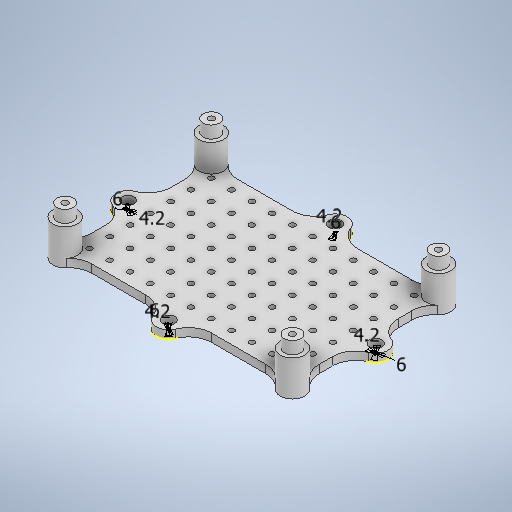
# Autodesk Inventor part: Bottom_Tip_Matrix
Saved by Autodesk Inventor 2025.1 (Build 291241000, 241)
## iProperties
Created: 2025-02-14
Part Number: Bottom_Tip_Matrix
Material: Generic
Document SubType Name: Modeling
Designer: m_kni
Density: 1 g/cm^3
Appearance: Default
Author: m_kni
Autodesk Inventor part; units mm, degrees
ref_plane "YZ Plane" through (0, 0, 0) normal (1, 0, 0) x (0, 1, 0)
ref_plane "XZ Plane" through (0, 0, 0) normal (0, 1, 0) x (-1, 0, 0)
ref_plane "XY Plane" through (0, 0, 0) normal (0, 0, 1) x (1, 0, 0)
sketch "Sketch1" plane through (0, 0, 0) normal (0, 1, 0) x (-1, 0, 0)
  line L0 (54.0633, -35.7627) -> (-55.9367, -35.7627)
  line L1 (-55.9367, -35.7627) -> (-55.9367, 36.2373)
  line L2 (-55.9367, 36.2373) -> (54.0633, 36.2373)
  line L3 (54.0633, -35.7627) -> (-55.9367, 36.2373) construction
  line L4 (-55.9367, -35.7627) -> (54.0633, 36.2373) construction
  circle A0 centre (-49.9367, 30.2373) radius 1.35
  circle A1 centre (-49.9367, 20.2373) radius 1.35
  circle A2 centre (-49.9367, 10.2373) radius 1.35
  circle A3 centre (-49.9367, 0.2373) radius 1.35
  circle A4 centre (-49.9367, -9.7627) radius 1.35
  circle A5 centre (-49.9367, -19.7627) radius 1.35
  circle A6 centre (-49.9367, -29.7627) radius 1.35
  circle A7 centre (-39.9367, 30.2373) radius 1.35
  circle A8 centre (-39.9367, 20.2373) radius 1.35
  circle A9 centre (-39.9367, 10.2373) radius 1.35
  circle A10 centre (-39.9367, 0.2373) radius 1.35
  circle A11 centre (-39.9367, -9.7627) radius 1.35
  circle A12 centre (-39.9367, -19.7627) radius 1.35
  circle A13 centre (-39.9367, -29.7627) radius 1.35
  circle A14 centre (-29.9367, 30.2373) radius 1.35
  circle A15 centre (-29.9367, 20.2373) radius 1.35
  circle A16 centre (-29.9367, 10.2373) radius 1.35
  circle A17 centre (-29.9367, 0.2373) radius 1.35
  circle A18 centre (-29.9367, -9.7627) radius 1.35
  circle A19 centre (-29.9367, -19.7627) radius 1.35
  circle A20 centre (-29.9367, -29.7627) radius 1.35
  circle A21 centre (-19.9367, 30.2373) radius 1.35
  circle A22 centre (-19.9367, 20.2373) radius 1.35
  circle A23 centre (-19.9367, 10.2373) radius 1.35
  circle A24 centre (-19.9367, 0.2373) radius 1.35
  circle A25 centre (-19.9367, -9.7627) radius 1.35
  circle A26 centre (-19.9367, -19.7627) radius 1.35
  circle A27 centre (-19.9367, -29.7627) radius 1.35
  circle A28 centre (-9.9367, 30.2373) radius 1.35
  circle A29 centre (-9.9367, 20.2373) radius 1.35
  circle A30 centre (-9.9367, 10.2373) radius 1.35
  circle A31 centre (-9.9367, 0.2373) radius 1.35
  circle A32 centre (-9.9367, -9.7627) radius 1.35
  circle A33 centre (-9.9367, -19.7627) radius 1.35
  circle A34 centre (-9.9367, -29.7627) radius 1.35
  circle A35 centre (0.0633, 30.2373) radius 1.35
  circle A36 centre (0.0633, 20.2373) radius 1.35
  circle A37 centre (0.0633, 10.2373) radius 1.35
  circle A38 centre (0.0633, 0.2373) radius 1.35
  circle A39 centre (0.0633, -9.7627) radius 1.35
  circle A40 centre (0.0633, -19.7627) radius 1.35
  circle A41 centre (0.0633, -29.7627) radius 1.35
  circle A42 centre (10.0633, 30.2373) radius 1.35
  circle A43 centre (10.0633, 20.2373) radius 1.35
  circle A44 centre (10.0633, 10.2373) radius 1.35
  circle A45 centre (10.0633, 0.2373) radius 1.35
  circle A46 centre (10.0633, -9.7627) radius 1.35
  circle A47 centre (10.0633, -19.7627) radius 1.35
  circle A48 centre (10.0633, -29.7627) radius 1.35
  circle A49 centre (20.0633, 30.2373) radius 1.35
  circle A50 centre (20.0633, 20.2373) radius 1.35
  circle A51 centre (20.0633, 10.2373) radius 1.35
  circle A52 centre (20.0633, 0.2373) radius 1.35
  circle A53 centre (20.0633, -9.7627) radius 1.35
  circle A54 centre (20.0633, -19.7627) radius 1.35
  circle A55 centre (20.0633, -29.7627) radius 1.35
  circle A56 centre (30.0633, 30.2373) radius 1.35
  circle A57 centre (30.0633, 20.2373) radius 1.35
  circle A58 centre (30.0633, 10.2373) radius 1.35
  circle A59 centre (30.0633, 0.2373) radius 1.35
  circle A60 centre (30.0633, -9.7627) radius 1.35
  circle A61 centre (30.0633, -19.7627) radius 1.35
  circle A62 centre (30.0633, -29.7627) radius 1.35
  circle A63 centre (40.0633, 30.2373) radius 1.35
  circle A64 centre (40.0633, 20.2373) radius 1.35
  circle A65 centre (40.0633, 10.2373) radius 1.35
  circle A66 centre (40.0633, 0.2373) radius 1.35
  circle A67 centre (40.0633, -9.7627) radius 1.35
  circle A68 centre (40.0633, -19.7627) radius 1.35
  circle A69 centre (40.0633, -29.7627) radius 1.35
  circle A70 centre (50.0633, 30.2373) radius 1.35
  circle A71 centre (50.0633, 20.2373) radius 1.35
  circle A72 centre (50.0633, 10.2373) radius 1.35
  circle A73 centre (50.0633, 0.2373) radius 1.35
  circle A74 centre (50.0633, -9.7627) radius 1.35
  circle A75 centre (50.0633, -19.7627) radius 1.35
  circle A76 centre (50.0633, -29.7627) radius 1.35
  line L5 (-55.9367, 36.2373) -> (56.0633, 36.2373)
  line L6 (56.0633, 36.2373) -> (56.0633, -35.7627)
  line L7 (56.0633, -35.7627) -> (-55.9367, -35.7627)
  line L8 (-55.9367, -35.7627) -> (-55.9367, 36.2373)
  circle A77 centre (-55.9367, 36.2373) radius 6
  circle A78 centre (-55.9367, -35.7627) radius 6
  circle A79 centre (56.0633, 36.2373) radius 6
  circle A80 centre (56.0633, -35.7627) radius 6
  point P0 (0, 0)
  point P1 (-0.9367, 0.2373)
  point P2 (56.0633, 30.2373)
  point P3 (-49.9367, -35.7627)
  point P4 (56.0633, -29.7627)
  point P5 (56.0633, 30.2373)
  point P6 (50.0633, 36.2373)
  point P7 (-49.9367, 36.2373)
  point P8 (-55.9367, 30.2373)
  point P9 (-55.9367, -29.7627)
  point P10 (-49.9367, -35.7627)
  point P11 (50.0633, -35.7627)
  dimension "d4" = 110
  dimension "d5" = 72
  dimension "d6" = 2.7
  dimension "d7" = 6
  dimension "d8" = 6
  dimension "d9" = 10
  dimension "d10" = 10
  dimension "d11" = 6
  dimension "d12" = 6
  dimension "d13" = 12
  dimension "d14" = 12
  dimension "d15" = 12
  dimension "d16" = 12
  constraints: 81 centre point, 18 end point, 5 coincident, 3 horizontal, 3 parallel, 2 midpoint, 2 perpendicular, 1 vertical, 152 other
  measures "d4" distance of L1.end L4.end
  measures "d5" distance of L1.start L1.end
  measures "d6" diameter of A0
  measures "d7" distance from line of A0.centre L2
  measures "d8" distance from line of A0.centre L1
  measures "d9" distance of A0.centre A1.centre
  measures "d10" distance of A0.centre A7.centre
  measures "d11" distance of point (56.063, 30.237) A70.centre
  measures "d12" distance of point (-49.937, -35.763) A6.centre
  measures "d13" diameter of A77
  measures "d14" diameter of A78
  measures "d15" diameter of A79
  measures "d16" diameter of A80
extrude "Extrusion1" add sketch "Sketch1" along normal blind 4
sketch "Sketch2" plane through (0, 4, 0) normal (0, 1, 0) x (1, 0, 0)
  arc A0 (49.9367, -36.2373) -> (55.9367, -30.2373) centre (55.9367, -36.2373) ccw projected
  arc A1 (-56.0633, -30.2373) -> (-50.0633, -36.2373) centre (-56.0633, -36.2373) ccw projected
  arc A2 (-50.0633, 35.7627) -> (-56.0633, 29.7627) centre (-56.0633, 35.7627) ccw projected
  arc A3 (55.9367, 29.7627) -> (49.9367, 35.7627) centre (55.9367, 35.7627) ccw projected
  circle A4 centre (-56.0633, -36.2373) radius 6
  circle A5 centre (-56.0633, 35.7627) radius 6
  circle A6 centre (55.9367, -36.2373) radius 6
  circle A7 centre (55.9367, 35.7627) radius 6
  point P0 (0, 0)
  point P1 (55.9367, 29.7627)
  point P2 (-56.0633, 29.7627)
  constraints: 4 coincident, 3 centre point, 3 concentric, 3 other
extrude "Extrusion2" add sketch "Sketch2" along normal blind 13.5
sketch "Sketch3" plane through (55.9367, 17.5, 36.2373) normal (0, 1, 0) x (1, 0, 0)
  circle A0 centre (0, 0) radius 4
  arc A1 (0, 66) -> (-6, 72) centre (0, 72) ccw projected
  circle A2 centre (0, 72) radius 4
  arc A3 (-112, 6) -> (-106, 0) centre (-112, 0) ccw projected
  circle A4 centre (-112, 0) radius 4
  circle A5 centre (-112, 72) radius 4
  point P0 (-55.9367, 36.2373)
  dimension "d21" = 8
  dimension "d22" = 8
  dimension "d23" = 8
  dimension "d24" = 8
  constraints: 4 centre point, 2 coincident
  measures "d21" diameter of A0
  measures "d22" diameter of A2
  measures "d23" diameter of A4
  measures "d24" diameter of A5
extrude "Extrusion3" add sketch "Sketch3" along normal blind 6
sketch "Sketch4" plane through (-56.0633, 23.5, 36.2373) normal (0, 1, 0) x (1, 0, 0)
  circle A0 centre (0, 0) radius 4 projected
  circle A1 centre (0, 72) radius 4 projected
  circle A2 centre (112, 0) radius 4 projected
  circle A3 centre (112, 72) radius 4 projected
  circle A4 centre (0, 0) radius 1.5
  circle A5 centre (112, 0) radius 1.5
  circle A6 centre (0, 72) radius 1.5
  circle A7 centre (112, 72) radius 1.5
  point P0 (56.0633, 36.2373)
  dimension "d27" = 3
  dimension "d28" = 3
  dimension "d29" = 3
  dimension "d30" = 3
  constraints: 4 centre point, 4 coincident
  measures "d27" diameter of A4
  measures "d28" diameter of A5
  measures "d29" diameter of A6
  measures "d30" diameter of A7
extrude "Extrusion4" cut sketch "Sketch4" against normal blind 8 contours A4 | A5 | A6 | A7
sketch "Sketch5" plane through (0, 4, 0) normal (0, 1, 0) x (1, 0, 0)
  line L0 (-50.0633, -36.2373) -> (49.9367, -36.2373) projected
  line L1 (-0.0633, -36.2373) -> (-0.0633, -41.2373)
  circle A0 centre (-0.0633, -41.2373) radius 6
  line L2 (49.9367, 35.7627) -> (-50.0633, 35.7627) projected
  line L3 (-56.0633, 29.7627) -> (-56.0633, -30.2373) projected
  line L4 (55.9367, -30.2373) -> (55.9367, 29.7627) projected
  circle A1 centre (60.9367, -0.2373) radius 6
  circle A2 centre (-0.0633, 40.7627) radius 6
  circle A3 centre (-61.0633, -0.2373) radius 6
  line L5 (60.9367, -6.2373) -> (55.9367, -6.2373)
  line L6 (60.9367, 5.7627) -> (55.9367, 5.7627)
  line L7 (-61.0633, 5.7627) -> (-56.0633, 5.7627)
  line L8 (-61.0633, -6.2373) -> (-56.0633, -6.2373)
  line L9 (-6.0633, -41.2373) -> (-6.0633, -36.2373)
  line L10 (5.9367, -41.2373) -> (5.9367, -36.2373)
  line L11 (-6.0633, 40.7627) -> (-6.0633, 35.7627)
  line L12 (5.9367, 40.7627) -> (5.9367, 35.7627)
  line L13 (-6.0633, -36.2373) -> (-5.0805, -36.2373)
  circle A4 centre (49.9367, -10.2373) radius 1.35 projected
  circle A5 centre (49.9367, -0.2373) radius 1.35 projected
  circle A6 centre (39.9367, -10.2373) radius 1.35 projected
  circle A7 centre (39.9367, -30.2373) radius 1.35 projected
  circle A8 centre (39.9367, -10.2373) radius 1.35 projected
  circle A9 centre (39.9367, 9.7627) radius 1.35 projected
  circle A10 centre (39.9367, 9.7627) radius 1.35 projected
  circle A11 centre (39.9367, 9.7627) radius 1.35 projected
  circle A12 centre (39.9367, 9.7627) radius 1.35 projected
  circle A13 centre (39.9367, 19.7627) radius 1.35 projected
  circle A14 centre (49.9367, 9.7627) radius 1.35 projected
  arc A15 (49.9367, -36.2373) -> (55.9367, -30.2373) centre (55.9367, -36.2373) ccw projected
  arc A16 (55.9367, -30.2373) -> (49.9367, -36.2373) centre (55.9367, -36.2373) ccw projected
  arc A17 (49.9367, 35.7627) -> (55.9367, 29.7627) centre (55.9367, 35.7627) ccw projected
  circle A18 centre (9.9367, 19.7627) radius 1.35 projected
  circle A19 centre (9.9367, 19.7627) radius 1.35 projected
  circle A20 centre (55.9367, 35.7627) radius 4 projected
  circle A21 centre (55.9367, 35.7627) radius 1.5 projected
  circle A22 centre (55.9367, 35.7627) radius 1.5 projected
  circle A23 centre (55.9367, 35.7627) radius 1.5 projected
  circle A24 centre (55.9367, 35.7627) radius 4 projected
  circle A25 centre (55.9367, 35.7627) radius 1.5 projected
  circle A26 centre (55.9367, 35.7627) radius 1.5 projected
  circle A27 centre (55.9367, 35.7627) radius 1.5 projected
  circle A28 centre (9.9367, 29.7627) radius 1.35 projected
  circle A29 centre (9.9367, 29.7627) radius 1.35 projected
  circle A30 centre (9.9367, 29.7627) radius 1.35 projected
  circle A31 centre (9.9367, 29.7627) radius 1.35 projected
  circle A32 centre (19.9367, 29.7627) radius 1.35 projected
  circle A33 centre (19.9367, 29.7627) radius 1.35 projected
  circle A34 centre (19.9367, 9.7627) radius 1.35 projected
  circle A35 centre (19.9367, 9.7627) radius 1.35 projected
  circle A36 centre (19.9367, 9.7627) radius 1.35 projected
  circle A37 centre (19.9367, 9.7627) radius 1.35 projected
  circle A38 centre (19.9367, 19.7627) radius 1.35 projected
  circle A39 centre (19.9367, 19.7627) radius 1.35 projected
  circle A40 centre (19.9367, 19.7627) radius 1.35 projected
  circle A41 centre (19.9367, 29.7627) radius 1.35 projected
  circle A42 centre (19.9367, 29.7627) radius 1.35 projected
  circle A43 centre (9.9367, 9.7627) radius 1.35 projected
  circle A44 centre (9.9367, 9.7627) radius 1.35 projected
  circle A45 centre (9.9367, 19.7627) radius 1.35 projected
  circle A46 centre (9.9367, 19.7627) radius 1.35 projected
  circle A47 centre (9.9367, 9.7627) radius 1.35 projected
  circle A48 centre (19.9367, 19.7627) radius 1.35 projected
  circle A49 centre (29.9367, 29.7627) radius 1.35 projected
  arc A50 (55.9367, 29.7627) -> (49.9367, 35.7627) centre (55.9367, 35.7627) ccw projected
  circle A51 centre (29.9367, 9.7627) radius 1.35 projected
  circle A52 centre (-0.0633, -0.2373) radius 1.35 projected
  circle A53 centre (-0.0633, -0.2373) radius 1.35 projected
  circle A54 centre (-0.0633, -10.2373) radius 1.35 projected
  circle A55 centre (-10.0633, -10.2373) radius 1.35 projected
  circle A56 centre (-10.0633, -10.2373) radius 1.35 projected
  circle A57 centre (55.9367, -36.2373) radius 1.5 projected
  circle A58 centre (49.9367, 9.7627) radius 1.35 projected
  circle A59 centre (49.9367, 9.7627) radius 1.35 projected
  circle A60 centre (55.9367, -36.2373) radius 4 projected
  circle A61 centre (49.9367, 19.7627) radius 1.35 projected
  circle A62 centre (49.9367, 19.7627) radius 1.35 projected
  circle A63 centre (-0.0633, 9.7627) radius 1.35 projected
  circle A64 centre (-10.0633, 9.7627) radius 1.35 projected
  circle A65 centre (-10.0633, 9.7627) radius 1.35 projected
  circle A66 centre (-0.0633, 9.7627) radius 1.35 projected
  circle A67 centre (-0.0633, -20.2373) radius 1.35 projected
  circle A68 centre (-0.0633, -20.2373) radius 1.35 projected
  circle A69 centre (19.9367, -20.2373) radius 1.35 projected
  circle A70 centre (9.9367, -30.2373) radius 1.35 projected
  circle A71 centre (-0.0633, -30.2373) radius 1.35 projected
  circle A72 centre (-0.0633, -30.2373) radius 1.35 projected
  circle A73 centre (-10.0633, -20.2373) radius 1.35 projected
  circle A74 centre (-10.0633, -20.2373) radius 1.35 projected
  circle A75 centre (19.9367, -20.2373) radius 1.35 projected
  circle A76 centre (9.9367, -0.2373) radius 1.35 projected
  circle A77 centre (-10.0633, -30.2373) radius 1.35 projected
  circle A78 centre (-10.0633, -30.2373) radius 1.35 projected
  circle A79 centre (9.9367, -0.2373) radius 1.35 projected
  circle A80 centre (-0.0633, 19.7627) radius 1.35 projected
  circle A81 centre (-0.0633, 19.7627) radius 1.35 projected
  circle A82 centre (-0.0633, 29.7627) radius 1.35 projected
  circle A83 centre (-0.0633, 29.7627) radius 1.35 projected
  circle A84 centre (-10.0633, 19.7627) radius 1.35 projected
  circle A85 centre (-10.0633, 19.7627) radius 1.35 projected
  circle A86 centre (-0.0633, 19.7627) radius 1.35 projected
  circle A87 centre (-0.0633, 19.7627) radius 1.35 projected
  circle A88 centre (-0.0633, 29.7627) radius 1.35 projected
  circle A89 centre (-0.0633, 29.7627) radius 1.35 projected
  circle A90 centre (-10.0633, -0.2373) radius 1.35 projected
  circle A91 centre (-10.0633, -0.2373) radius 1.35 projected
  circle A92 centre (55.9367, -36.2373) radius 4 projected
  circle A93 centre (55.9367, -36.2373) radius 1.5 projected
  circle A94 centre (55.9367, -36.2373) radius 1.5 projected
  circle A95 centre (55.9367, -36.2373) radius 4 projected
  circle A96 centre (55.9367, -36.2373) radius 1.5 projected
  circle A97 centre (55.9367, -36.2373) radius 1.5 projected
  circle A98 centre (39.9367, -30.2373) radius 1.35 projected
  circle A99 centre (39.9367, -30.2373) radius 1.35 projected
  circle A100 centre (39.9367, -0.2373) radius 1.35 projected
  circle A101 centre (39.9367, -0.2373) radius 1.35 projected
  circle A102 centre (39.9367, -10.2373) radius 1.35 projected
  circle A103 centre (39.9367, -10.2373) radius 1.35 projected
  circle A104 centre (39.9367, -20.2373) radius 1.35 projected
  circle A105 centre (39.9367, -20.2373) radius 1.35 projected
  circle A106 centre (49.9367, -20.2373) radius 1.35 projected
  circle A107 centre (49.9367, -20.2373) radius 1.35 projected
  circle A108 centre (49.9367, -10.2373) radius 1.35 projected
  circle A109 centre (49.9367, -10.2373) radius 1.35 projected
  circle A110 centre (49.9367, -30.2373) radius 1.35 projected
  circle A111 centre (49.9367, -30.2373) radius 1.35 projected
  circle A112 centre (55.9367, -36.2373) radius 4 projected
  circle A113 centre (55.9367, -36.2373) radius 4 projected
  circle A114 centre (55.9367, -36.2373) radius 6 projected
  circle A115 centre (55.9367, -36.2373) radius 6 projected
  arc A116 (49.9367, -36.2373) -> (55.9367, -30.2373) centre (55.9367, -36.2373) ccw projected
  arc A117 (55.9367, -30.2373) -> (49.9367, -36.2373) centre (55.9367, -36.2373) ccw projected
  circle A118 centre (55.9367, -36.2373) radius 4 projected
  circle A119 centre (55.9367, -36.2373) radius 6 projected
  line L14 (55.9367, -30.2373) -> (55.9367, 29.7627) projected
  line L15 (55.9367, -30.2373) -> (55.9367, 29.7627) projected
  circle A120 centre (49.9367, -0.2373) radius 1.35 projected
  circle A121 centre (49.9367, -0.2373) radius 1.35 projected
  circle A122 centre (-20.0633, 19.7627) radius 1.35 projected
  circle A123 centre (-20.0633, 29.7627) radius 1.35 projected
  circle A124 centre (-20.0633, 29.7627) radius 1.35 projected
  circle A125 centre (-20.0633, 19.7627) radius 1.35 projected
  circle A126 centre (-40.0633, -20.2373) radius 1.35 projected
  circle A127 centre (-40.0633, -20.2373) radius 1.35 projected
  circle A128 centre (-40.0633, -30.2373) radius 1.35 projected
  circle A129 centre (-40.0633, -30.2373) radius 1.35 projected
  circle A130 centre (-30.0633, -20.2373) radius 1.35 projected
  circle A131 centre (-30.0633, -20.2373) radius 1.35 projected
  circle A132 centre (-20.0633, 9.7627) radius 1.35 projected
  circle A133 centre (-20.0633, 9.7627) radius 1.35 projected
  circle A134 centre (-30.0633, -0.2373) radius 1.35 projected
  circle A135 centre (-30.0633, -0.2373) radius 1.35 projected
  circle A136 centre (-20.0633, -30.2373) radius 1.35 projected
  circle A137 centre (-20.0633, -30.2373) radius 1.35 projected
  circle A138 centre (-20.0633, -10.2373) radius 1.35 projected
  circle A139 centre (-20.0633, -10.2373) radius 1.35 projected
  circle A140 centre (-20.0633, -0.2373) radius 1.35 projected
  circle A141 centre (-20.0633, -0.2373) radius 1.35 projected
  circle A142 centre (-30.0633, 9.7627) radius 1.35 projected
  circle A143 centre (-20.0633, -20.2373) radius 1.35 projected
  circle A144 centre (-20.0633, -20.2373) radius 1.35 projected
  circle A145 centre (-30.0633, -10.2373) radius 1.35 projected
  circle A146 centre (-30.0633, -10.2373) radius 1.35 projected
  circle A147 centre (-40.0633, -10.2373) radius 1.35 projected
  circle A148 centre (-30.0633, -30.2373) radius 1.35 projected
  circle A149 centre (-30.0633, -30.2373) radius 1.35 projected
  circle A150 centre (-30.0633, 9.7627) radius 1.35 projected
  circle A151 centre (-40.0633, -0.2373) radius 1.35 projected
  circle A152 centre (-40.0633, -0.2373) radius 1.35 projected
  circle A153 centre (-50.0633, 19.7627) radius 1.35 projected
  circle A154 centre (-50.0633, 19.7627) radius 1.35 projected
  circle A155 centre (-50.0633, 9.7627) radius 1.35 projected
  circle A156 centre (-50.0633, 9.7627) radius 1.35 projected
  circle A157 centre (-40.0633, 19.7627) radius 1.35 projected
  circle A158 centre (-40.0633, 19.7627) radius 1.35 projected
  circle A159 centre (-50.0633, -10.2373) radius 1.35 projected
  circle A160 centre (-30.0633, 19.7627) radius 1.35 projected
  circle A161 centre (-30.0633, 29.7627) radius 1.35 projected
  circle A162 centre (-30.0633, 29.7627) radius 1.35 projected
  circle A163 centre (-50.0633, -10.2373) radius 1.35 projected
  circle A164 centre (-30.0633, 19.7627) radius 1.35 projected
  circle A165 centre (-56.0633, -36.2373) radius 1.5 projected
  circle A166 centre (-56.0633, -36.2373) radius 1.5 projected
  circle A167 centre (-56.0633, -36.2373) radius 1.5 projected
  circle A168 centre (-56.0633, -36.2373) radius 1.5 projected
  circle A169 centre (-56.0633, -36.2373) radius 1.5 projected
  arc A170 (-50.0633, -36.2373) -> (-56.0633, -30.2373) centre (-56.0633, -36.2373) ccw projected
  arc A171 (-56.0633, -30.2373) -> (-50.0633, -36.2373) centre (-56.0633, -36.2373) ccw projected
  line L16 (-56.0633, 29.7627) -> (-56.0633, -30.2373) projected
  arc A172 (-56.0633, 29.7627) -> (-50.0633, 35.7627) centre (-56.0633, 35.7627) ccw projected
  arc A173 (-50.0633, 35.7627) -> (-56.0633, 29.7627) centre (-56.0633, 35.7627) ccw projected
  circle A174 centre (-56.0633, 35.7627) radius 4 projected
  circle A175 centre (-56.0633, 35.7627) radius 1.5 projected
  circle A176 centre (-56.0633, 35.7627) radius 1.5 projected
  circle A177 centre (-56.0633, 35.7627) radius 1.5 projected
  circle A178 centre (-56.0633, 35.7627) radius 4 projected
  circle A179 centre (-56.0633, 35.7627) radius 1.5 projected
  circle A180 centre (-56.0633, 35.7627) radius 1.5 projected
  circle A181 centre (-56.0633, 35.7627) radius 6 projected
  arc A182 (-50.0633, 35.7627) -> (-56.0633, 29.7627) centre (-56.0633, 35.7627) ccw projected
  arc A183 (-56.0633, 29.7627) -> (-50.0633, 35.7627) centre (-56.0633, 35.7627) ccw projected
  circle A184 centre (-50.0633, 19.7627) radius 1.35 projected
  circle A185 centre (-50.0633, 19.7627) radius 1.35 projected
  circle A186 centre (-50.0633, 9.7627) radius 1.35 projected
  circle A187 centre (-50.0633, 9.7627) radius 1.35 projected
  circle A188 centre (-40.0633, 19.7627) radius 1.35 projected
  circle A189 centre (-40.0633, 19.7627) radius 1.35 projected
  circle A190 centre (-10.0633, 9.7627) radius 1.35 projected
  circle A191 centre (-10.0633, 9.7627) radius 1.35 projected
  circle A192 centre (-30.0633, 9.7627) radius 1.35 projected
  circle A193 centre (-30.0633, 9.7627) radius 1.35 projected
  circle A194 centre (-40.0633, 9.7627) radius 1.35 projected
  circle A195 centre (-40.0633, 9.7627) radius 1.35 projected
  circle A196 centre (-30.0633, 19.7627) radius 1.35 projected
  circle A197 centre (-30.0633, 19.7627) radius 1.35 projected
  circle A198 centre (-56.0633, 35.7627) radius 4 projected
  circle A199 centre (-56.0633, 35.7627) radius 4 projected
  circle A200 centre (-56.0633, 35.7627) radius 4 projected
  circle A201 centre (-56.0633, 35.7627) radius 6 projected
  circle A202 centre (-50.0633, 29.7627) radius 1.35 projected
  circle A203 centre (-50.0633, 29.7627) radius 1.35 projected
  circle A204 centre (-20.0633, 19.7627) radius 1.35 projected
  circle A205 centre (-20.0633, 19.7627) radius 1.35 projected
  circle A206 centre (-40.0633, 29.7627) radius 1.35 projected
  circle A207 centre (-40.0633, 29.7627) radius 1.35 projected
  circle A208 centre (-30.0633, 29.7627) radius 1.35 projected
  circle A209 centre (-30.0633, 29.7627) radius 1.35 projected
  circle A210 centre (-10.0633, 19.7627) radius 1.35 projected
  circle A211 centre (-10.0633, 19.7627) radius 1.35 projected
  circle A212 centre (-20.0633, 29.7627) radius 1.35 projected
  circle A213 centre (-20.0633, 29.7627) radius 1.35 projected
  circle A214 centre (-10.0633, 29.7627) radius 1.35 projected
  circle A215 centre (-10.0633, 29.7627) radius 1.35 projected
  circle A216 centre (-20.0633, 9.7627) radius 1.35 projected
  circle A217 centre (-20.0633, 9.7627) radius 1.35 projected
  circle A218 centre (-56.0633, -36.2373) radius 4 projected
  circle A219 centre (-56.0633, -36.2373) radius 1.5 projected
  circle A220 centre (-56.0633, -36.2373) radius 4 projected
  circle A221 centre (-56.0633, -36.2373) radius 4 projected
  circle A222 centre (-56.0633, -36.2373) radius 6 projected
  arc A223 (-56.0633, -30.2373) -> (-50.0633, -36.2373) centre (-56.0633, -36.2373) ccw projected
  arc A224 (-50.0633, -36.2373) -> (-56.0633, -30.2373) centre (-56.0633, -36.2373) ccw projected
  line L17 (-56.0633, 29.7627) -> (-56.0633, -30.2373) projected
  line L18 (-56.0633, 29.7627) -> (-56.0633, -30.2373) projected
  circle A225 centre (-40.0633, -0.2373) radius 1.35 projected
  circle A226 centre (-40.0633, -0.2373) radius 1.35 projected
  circle A227 centre (-50.0633, -10.2373) radius 1.35 projected
  circle A228 centre (-50.0633, -10.2373) radius 1.35 projected
  circle A229 centre (-40.0633, -20.2373) radius 1.35 projected
  circle A230 centre (-40.0633, -20.2373) radius 1.35 projected
  circle A231 centre (-40.0633, -30.2373) radius 1.35 projected
  circle A232 centre (-40.0633, -30.2373) radius 1.35 projected
  circle A233 centre (-30.0633, -20.2373) radius 1.35 projected
  circle A234 centre (-30.0633, -20.2373) radius 1.35 projected
  circle A235 centre (-30.0633, -0.2373) radius 1.35 projected
  circle A236 centre (-30.0633, -0.2373) radius 1.35 projected
  circle A237 centre (-10.0633, -0.2373) radius 1.35 projected
  circle A238 centre (-10.0633, -0.2373) radius 1.35 projected
  circle A239 centre (-20.0633, -0.2373) radius 1.35 projected
  circle A240 centre (-20.0633, -0.2373) radius 1.35 projected
  circle A241 centre (-50.0633, -0.2373) radius 1.35 projected
  circle A242 centre (-50.0633, -0.2373) radius 1.35 projected
  circle A243 centre (-20.0633, -10.2373) radius 1.35 projected
  circle A244 centre (-20.0633, -10.2373) radius 1.35 projected
  circle A245 centre (-10.0633, -10.2373) radius 1.35 projected
  circle A246 centre (-10.0633, -10.2373) radius 1.35 projected
  circle A247 centre (-40.0633, -10.2373) radius 1.35 projected
  circle A248 centre (-40.0633, -10.2373) radius 1.35 projected
  circle A249 centre (-10.0633, -20.2373) radius 1.35 projected
  circle A250 centre (-10.0633, -20.2373) radius 1.35 projected
  circle A251 centre (-20.0633, -20.2373) radius 1.35 projected
  circle A252 centre (-20.0633, -20.2373) radius 1.35 projected
  circle A253 centre (-10.0633, -30.2373) radius 1.35 projected
  circle A254 centre (-10.0633, -30.2373) radius 1.35 projected
  circle A255 centre (-20.0633, -30.2373) radius 1.35 projected
  circle A256 centre (-20.0633, -30.2373) radius 1.35 projected
  circle A257 centre (-30.0633, -30.2373) radius 1.35 projected
  circle A258 centre (-30.0633, -30.2373) radius 1.35 projected
  circle A259 centre (-50.0633, -20.2373) radius 1.35 projected
  circle A260 centre (-50.0633, -20.2373) radius 1.35 projected
  circle A261 centre (-50.0633, -30.2373) radius 1.35 projected
  circle A262 centre (-50.0633, -30.2373) radius 1.35 projected
  circle A263 centre (-56.0633, -36.2373) radius 4 projected
  circle A264 centre (-56.0633, -36.2373) radius 4 projected
  circle A265 centre (-56.0633, -36.2373) radius 4 projected
  circle A266 centre (-56.0633, -36.2373) radius 6 projected
  circle A267 centre (-30.0633, -10.2373) radius 1.35 projected
  circle A268 centre (-30.0633, -10.2373) radius 1.35 projected
  circle A269 centre (-40.0633, -10.2373) radius 1.35 projected
  circle A270 centre (-40.0633, 29.7627) radius 1.35 projected
  circle A271 centre (-40.0633, 29.7627) radius 1.35 projected
  circle A272 centre (-40.0633, 9.7627) radius 1.35 projected
  circle A273 centre (-50.0633, 29.7627) radius 1.35 projected
  circle A274 centre (-50.0633, 29.7627) radius 1.35 projected
  circle A275 centre (-56.0633, 35.7627) radius 4 projected
  circle A276 centre (-56.0633, 35.7627) radius 6 projected
  circle A277 centre (-50.0633, -0.2373) radius 1.35 projected
  circle A278 centre (-50.0633, -0.2373) radius 1.35 projected
  circle A279 centre (-50.0633, -20.2373) radius 1.35 projected
  circle A280 centre (-50.0633, -20.2373) radius 1.35 projected
  circle A281 centre (-50.0633, -30.2373) radius 1.35 projected
  circle A282 centre (-50.0633, -30.2373) radius 1.35 projected
  circle A283 centre (-56.0633, -36.2373) radius 6 projected
  circle A284 centre (-40.0633, 9.7627) radius 1.35 projected
  circle A285 centre (29.9367, 29.7627) radius 1.35 projected
  circle A286 centre (49.9367, -0.2373) radius 1.35 projected
  circle A287 centre (29.9367, 9.7627) radius 1.35 projected
  circle A288 centre (29.9367, 9.7627) radius 1.35 projected
  circle A289 centre (29.9367, 9.7627) radius 1.35 projected
  circle A290 centre (39.9367, -0.2373) radius 1.35 projected
  circle A291 centre (39.9367, -0.2373) radius 1.35 projected
  circle A292 centre (29.9367, -0.2373) radius 1.35 projected
  circle A293 centre (49.9367, -10.2373) radius 1.35 projected
  circle A294 centre (29.9367, -0.2373) radius 1.35 projected
  circle A295 centre (19.9367, -0.2373) radius 1.35 projected
  circle A296 centre (19.9367, -0.2373) radius 1.35 projected
  circle A297 centre (19.9367, -10.2373) radius 1.35 projected
  circle A298 centre (19.9367, -10.2373) radius 1.35 projected
  line L19 (55.9367, -30.2373) -> (55.9367, 29.7627) projected
  circle A299 centre (-10.0633, 29.7627) radius 1.35 projected
  circle A300 centre (-10.0633, 29.7627) radius 1.35 projected
  circle A301 centre (55.9367, -36.2373) radius 1.5 projected
  circle A302 centre (29.9367, -30.2373) radius 1.35 projected
  circle A303 centre (29.9367, -30.2373) radius 1.35 projected
  circle A304 centre (19.9367, -30.2373) radius 1.35 projected
  line L20 (49.9367, 35.7627) -> (-50.0633, 35.7627) projected
  line L21 (49.9367, 35.7627) -> (-50.0633, 35.7627) projected
  line L22 (49.9367, 35.7627) -> (-50.0633, 35.7627) projected
  circle A305 centre (-56.0633, 35.7627) radius 1.5 projected
  line L23 (-50.0633, -36.2373) -> (49.9367, -36.2373) projected
  line L24 (-50.0633, -36.2373) -> (49.9367, -36.2373) projected
  line L25 (-50.0633, -36.2373) -> (49.9367, -36.2373) projected
  arc A306 (55.9367, -30.2373) -> (49.9367, -36.2373) centre (55.9367, -36.2373) ccw projected
  line L26 (55.9367, -30.2373) -> (55.9367, 29.7627) projected
  arc A307 (49.9367, 35.7627) -> (55.9367, 29.7627) centre (55.9367, 35.7627) ccw projected
  line L27 (49.9367, 35.7627) -> (-50.0633, 35.7627) projected
  arc A308 (-56.0633, 29.7627) -> (-50.0633, 35.7627) centre (-56.0633, 35.7627) ccw projected
  line L28 (-56.0633, 29.7627) -> (-56.0633, -30.2373) projected
  arc A309 (-50.0633, -36.2373) -> (-56.0633, -30.2373) centre (-56.0633, -36.2373) ccw projected
  line L29 (-50.0633, -36.2373) -> (49.9367, -36.2373) projected
  circle A310 centre (-40.0633, -0.2373) radius 1.35 projected
  circle A311 centre (-50.0633, 19.7627) radius 1.35 projected
  circle A312 centre (-50.0633, 9.7627) radius 1.35 projected
  circle A313 centre (-40.0633, 19.7627) radius 1.35 projected
  circle A314 centre (-50.0633, -10.2373) radius 1.35 projected
  circle A315 centre (-40.0633, -20.2373) radius 1.35 projected
  circle A316 centre (-40.0633, -30.2373) radius 1.35 projected
  circle A317 centre (-30.0633, -20.2373) radius 1.35 projected
  circle A318 centre (-30.0633, 19.7627) radius 1.35 projected
  circle A319 centre (-30.0633, 29.7627) radius 1.35 projected
  circle A320 centre (-20.0633, 9.7627) radius 1.35 projected
  circle A321 centre (-30.0633, -0.2373) radius 1.35 projected
  circle A322 centre (-20.0633, -30.2373) radius 1.35 projected
  circle A323 centre (-20.0633, -10.2373) radius 1.35 projected
  circle A324 centre (9.9367, 29.7627) radius 1.35 projected
  circle A325 centre (29.9367, -10.2373) radius 1.35 projected
  circle A326 centre (29.9367, -30.2373) radius 1.35 projected
  circle A327 centre (19.9367, -0.2373) radius 1.35 projected
  circle A328 centre (19.9367, -10.2373) radius 1.35 projected
  circle A329 centre (29.9367, 29.7627) radius 1.35 projected
  circle A330 centre (19.9367, 29.7627) radius 1.35 projected
  circle A331 centre (19.9367, 9.7627) radius 1.35 projected
  circle A332 centre (9.9367, -20.2373) radius 1.35 projected
  circle A333 centre (9.9367, -10.2373) radius 1.35 projected
  circle A334 centre (-0.0633, 19.7627) radius 1.35 projected
  circle A335 centre (-0.0633, 29.7627) radius 1.35 projected
  circle A336 centre (-10.0633, 29.7627) radius 1.35 projected
  circle A337 centre (-10.0633, -30.2373) radius 1.35 projected
  circle A338 centre (39.9367, -30.2373) radius 1.35 projected
  circle A339 centre (49.9367, -20.2373) radius 1.35 projected
  circle A340 centre (9.9367, -0.2373) radius 1.35 projected
  circle A341 centre (-10.0633, 9.7627) radius 1.35 projected
  circle A342 centre (-0.0633, 9.7627) radius 1.35 projected
  circle A343 centre (19.9367, -30.2373) radius 1.35 projected
  circle A344 centre (49.9367, -10.2373) radius 1.35 projected
  circle A345 centre (29.9367, -0.2373) radius 1.35 projected
  circle A346 centre (49.9367, -0.2373) radius 1.35 projected
  circle A347 centre (39.9367, -0.2373) radius 1.35 projected
  circle A348 centre (49.9367, 9.7627) radius 1.35 projected
  circle A349 centre (39.9367, 9.7627) radius 1.35 projected
  circle A350 centre (49.9367, 19.7627) radius 1.35 projected
  circle A351 centre (39.9367, 29.7627) radius 1.35 projected
  circle A352 centre (-0.0633, -0.2373) radius 1.35 projected
  circle A353 centre (-10.0633, -10.2373) radius 1.35 projected
  circle A354 centre (39.9367, 19.7627) radius 1.35 projected
  circle A355 centre (39.9367, -20.2373) radius 1.35 projected
  circle A356 centre (-10.0633, -20.2373) radius 1.35 projected
  circle A357 centre (-10.0633, 19.7627) radius 1.35 projected
  circle A358 centre (-10.0633, -0.2373) radius 1.35 projected
  circle A359 centre (-0.0633, -20.2373) radius 1.35 projected
  circle A360 centre (-0.0633, -30.2373) radius 1.35 projected
  circle A361 centre (-0.0633, -10.2373) radius 1.35 projected
  circle A362 centre (29.9367, 9.7627) radius 1.35 projected
  circle A363 centre (19.9367, 19.7627) radius 1.35 projected
  circle A364 centre (29.9367, 19.7627) radius 1.35 projected
  circle A365 centre (9.9367, -30.2373) radius 1.35 projected
  circle A366 centre (19.9367, -20.2373) radius 1.35 projected
  circle A367 centre (29.9367, -20.2373) radius 1.35 projected
  circle A368 centre (39.9367, -10.2373) radius 1.35 projected
  circle A369 centre (9.9367, 19.7627) radius 1.35 projected
  circle A370 centre (9.9367, 9.7627) radius 1.35 projected
  circle A371 centre (-20.0633, -20.2373) radius 1.35 projected
  circle A372 centre (-20.0633, -0.2373) radius 1.35 projected
  circle A373 centre (-30.0633, 9.7627) radius 1.35 projected
  circle A374 centre (-20.0633, 19.7627) radius 1.35 projected
  circle A375 centre (-20.0633, 29.7627) radius 1.35 projected
  circle A376 centre (-30.0633, -10.2373) radius 1.35 projected
  circle A377 centre (-30.0633, -30.2373) radius 1.35 projected
  circle A378 centre (-40.0633, -10.2373) radius 1.35 projected
  circle A379 centre (-50.0633, -20.2373) radius 1.35 projected
  circle A380 centre (-40.0633, 29.7627) radius 1.35 projected
  circle A381 centre (-40.0633, 9.7627) radius 1.35 projected
  circle A382 centre (-50.0633, -0.2373) radius 1.35 projected
  circle A383 centre (-50.0633, 29.7627) radius 1.35 projected
  circle A384 centre (-50.0633, -30.2373) radius 1.35 projected
  circle A385 centre (49.9367, -30.2373) radius 1.35 projected
  circle A386 centre (49.9367, 29.7627) radius 1.35 projected
  arc A387 (-56.0633, -30.2373) -> (-50.0633, -36.2373) centre (-56.0633, -36.2373) ccw projected
  line L30 (-56.0633, 29.7627) -> (-56.0633, -30.2373) projected
  arc A388 (-50.0633, 35.7627) -> (-56.0633, 29.7627) centre (-56.0633, 35.7627) ccw projected
  line L31 (49.9367, 35.7627) -> (-50.0633, 35.7627) projected
  arc A389 (55.9367, 29.7627) -> (49.9367, 35.7627) centre (55.9367, 35.7627) ccw projected
  line L32 (55.9367, -30.2373) -> (55.9367, 29.7627) projected
  arc A390 (49.9367, -36.2373) -> (55.9367, -30.2373) centre (55.9367, -36.2373) ccw projected
  line L33 (-50.0633, -36.2373) -> (49.9367, -36.2373) projected
  circle A391 centre (-40.0633, -0.2373) radius 1.35 projected
  circle A392 centre (-50.0633, 19.7627) radius 1.35 projected
  circle A393 centre (-50.0633, 9.7627) radius 1.35 projected
  circle A394 centre (-40.0633, 19.7627) radius 1.35 projected
  circle A395 centre (-50.0633, -10.2373) radius 1.35 projected
  circle A396 centre (-40.0633, -20.2373) radius 1.35 projected
  circle A397 centre (-40.0633, -30.2373) radius 1.35 projected
  circle A398 centre (-30.0633, -20.2373) radius 1.35 projected
  circle A399 centre (-30.0633, 19.7627) radius 1.35 projected
  circle A400 centre (-30.0633, 29.7627) radius 1.35 projected
  circle A401 centre (-20.0633, 9.7627) radius 1.35 projected
  circle A402 centre (-30.0633, -0.2373) radius 1.35 projected
  circle A403 centre (-20.0633, -30.2373) radius 1.35 projected
  circle A404 centre (-20.0633, -10.2373) radius 1.35 projected
  circle A405 centre (9.9367, 29.7627) radius 1.35 projected
  circle A406 centre (29.9367, -10.2373) radius 1.35 projected
  circle A407 centre (29.9367, -30.2373) radius 1.35 projected
  circle A408 centre (19.9367, -0.2373) radius 1.35 projected
  circle A409 centre (19.9367, -10.2373) radius 1.35 projected
  circle A410 centre (29.9367, 29.7627) radius 1.35 projected
  circle A411 centre (19.9367, 29.7627) radius 1.35 projected
  circle A412 centre (19.9367, 9.7627) radius 1.35 projected
  circle A413 centre (9.9367, -20.2373) radius 1.35 projected
  circle A414 centre (9.9367, -10.2373) radius 1.35 projected
  circle A415 centre (-0.0633, 19.7627) radius 1.35 projected
  circle A416 centre (-0.0633, 29.7627) radius 1.35 projected
  circle A417 centre (-10.0633, 29.7627) radius 1.35 projected
  circle A418 centre (-10.0633, -30.2373) radius 1.35 projected
  circle A419 centre (39.9367, -30.2373) radius 1.35 projected
  circle A420 centre (49.9367, -20.2373) radius 1.35 projected
  circle A421 centre (9.9367, -0.2373) radius 1.35 projected
  circle A422 centre (-10.0633, 9.7627) radius 1.35 projected
  circle A423 centre (-0.0633, 9.7627) radius 1.35 projected
  circle A424 centre (19.9367, -30.2373) radius 1.35 projected
  circle A425 centre (49.9367, -10.2373) radius 1.35 projected
  circle A426 centre (29.9367, -0.2373) radius 1.35 projected
  circle A427 centre (49.9367, -0.2373) radius 1.35 projected
  circle A428 centre (39.9367, -0.2373) radius 1.35 projected
  circle A429 centre (49.9367, 9.7627) radius 1.35 projected
  circle A430 centre (39.9367, 9.7627) radius 1.35 projected
  circle A431 centre (49.9367, 19.7627) radius 1.35 projected
  circle A432 centre (39.9367, 29.7627) radius 1.35 projected
  circle A433 centre (-0.0633, -0.2373) radius 1.35 projected
  circle A434 centre (-10.0633, -10.2373) radius 1.35 projected
  circle A435 centre (39.9367, 19.7627) radius 1.35 projected
  circle A436 centre (39.9367, -20.2373) radius 1.35 projected
  circle A437 centre (-10.0633, -20.2373) radius 1.35 projected
  circle A438 centre (-10.0633, 19.7627) radius 1.35 projected
  circle A439 centre (-10.0633, -0.2373) radius 1.35 projected
  circle A440 centre (-0.0633, -20.2373) radius 1.35 projected
  circle A441 centre (-0.0633, -30.2373) radius 1.35 projected
  circle A442 centre (-0.0633, -10.2373) radius 1.35 projected
  circle A443 centre (29.9367, 9.7627) radius 1.35 projected
  circle A444 centre (19.9367, 19.7627) radius 1.35 projected
  circle A445 centre (29.9367, 19.7627) radius 1.35 projected
  circle A446 centre (9.9367, -30.2373) radius 1.35 projected
  circle A447 centre (19.9367, -20.2373) radius 1.35 projected
  circle A448 centre (29.9367, -20.2373) radius 1.35 projected
  circle A449 centre (39.9367, -10.2373) radius 1.35 projected
  circle A450 centre (9.9367, 19.7627) radius 1.35 projected
  circle A451 centre (9.9367, 9.7627) radius 1.35 projected
  circle A452 centre (-20.0633, -20.2373) radius 1.35 projected
  circle A453 centre (-20.0633, -0.2373) radius 1.35 projected
  circle A454 centre (-30.0633, 9.7627) radius 1.35 projected
  circle A455 centre (-20.0633, 19.7627) radius 1.35 projected
  circle A456 centre (-20.0633, 29.7627) radius 1.35 projected
  circle A457 centre (-30.0633, -10.2373) radius 1.35 projected
  circle A458 centre (-30.0633, -30.2373) radius 1.35 projected
  circle A459 centre (-40.0633, -10.2373) radius 1.35 projected
  circle A460 centre (-50.0633, -20.2373) radius 1.35 projected
  circle A461 centre (-40.0633, 29.7627) radius 1.35 projected
  circle A462 centre (-40.0633, 9.7627) radius 1.35 projected
  circle A463 centre (-50.0633, -0.2373) radius 1.35 projected
  circle A464 centre (-50.0633, 29.7627) radius 1.35 projected
  circle A465 centre (-50.0633, -30.2373) radius 1.35 projected
  circle A466 centre (49.9367, -30.2373) radius 1.35 projected
  circle A467 centre (49.9367, 29.7627) radius 1.35 projected
  circle A468 centre (29.9367, -10.2373) radius 1.35 projected
  circle A469 centre (19.9367, -30.2373) radius 1.35 projected
  circle A470 centre (9.9367, -30.2373) radius 1.35 projected
  circle A471 centre (-0.0633, -10.2373) radius 1.35 projected
  circle A472 centre (9.9367, 9.7627) radius 1.35 projected
  circle A473 centre (29.9367, -10.2373) radius 1.35 projected
  circle A474 centre (9.9367, -20.2373) radius 1.35 projected
  circle A475 centre (9.9367, -20.2373) radius 1.35 projected
  circle A476 centre (29.9367, -10.2373) radius 1.35 projected
  circle A477 centre (29.9367, -10.2373) radius 1.35 projected
  circle A478 centre (29.9367, -30.2373) radius 1.35 projected
  circle A479 centre (29.9367, -30.2373) radius 1.35 projected
  circle A480 centre (29.9367, -0.2373) radius 1.35 projected
  circle A481 centre (29.9367, -0.2373) radius 1.35 projected
  circle A482 centre (29.9367, -20.2373) radius 1.35 projected
  circle A483 centre (29.9367, -20.2373) radius 1.35 projected
  circle A484 centre (19.9367, -0.2373) radius 1.35 projected
  circle A485 centre (19.9367, -0.2373) radius 1.35 projected
  circle A486 centre (19.9367, -10.2373) radius 1.35 projected
  circle A487 centre (19.9367, -10.2373) radius 1.35 projected
  circle A488 centre (19.9367, -20.2373) radius 1.35 projected
  circle A489 centre (19.9367, -20.2373) radius 1.35 projected
  circle A490 centre (19.9367, -30.2373) radius 1.35 projected
  circle A491 centre (19.9367, -30.2373) radius 1.35 projected
  circle A492 centre (9.9367, -10.2373) radius 1.35 projected
  circle A493 centre (9.9367, -20.2373) radius 1.35 projected
  circle A494 centre (9.9367, -20.2373) radius 1.35 projected
  circle A495 centre (9.9367, -10.2373) radius 1.35 projected
  circle A496 centre (9.9367, -10.2373) radius 1.35 projected
  circle A497 centre (9.9367, -0.2373) radius 1.35 projected
  circle A498 centre (9.9367, -0.2373) radius 1.35 projected
  circle A499 centre (-0.0633, 9.7627) radius 1.35 projected
  circle A500 centre (-0.0633, 9.7627) radius 1.35 projected
  circle A501 centre (-0.0633, -0.2373) radius 1.35 projected
  circle A502 centre (-0.0633, -0.2373) radius 1.35 projected
  circle A503 centre (9.9367, -30.2373) radius 1.35 projected
  circle A504 centre (9.9367, -30.2373) radius 1.35 projected
  circle A505 centre (-0.0633, -10.2373) radius 1.35 projected
  circle A506 centre (-0.0633, -10.2373) radius 1.35 projected
  circle A507 centre (-0.0633, -20.2373) radius 1.35 projected
  circle A508 centre (-0.0633, -20.2373) radius 1.35 projected
  circle A509 centre (-0.0633, -30.2373) radius 1.35 projected
  circle A510 centre (-0.0633, -30.2373) radius 1.35 projected
  circle A511 centre (9.9367, -10.2373) radius 1.35 projected
  circle A512 centre (49.9367, -20.2373) radius 1.35 projected
  circle A513 centre (49.9367, -20.2373) radius 1.35 projected
  circle A514 centre (39.9367, -20.2373) radius 1.35 projected
  circle A515 centre (39.9367, -20.2373) radius 1.35 projected
  circle A516 centre (39.9367, -30.2373) radius 1.35 projected
  circle A517 centre (29.9367, -20.2373) radius 1.35 projected
  circle A518 centre (49.9367, -30.2373) radius 1.35 projected
  circle A519 centre (49.9367, -30.2373) radius 1.35 projected
  circle A520 centre (29.9367, -20.2373) radius 1.35 projected
  circle A521 centre (29.9367, 19.7627) radius 1.35 projected
  circle A522 centre (39.9367, 19.7627) radius 1.35 projected
  circle A523 centre (39.9367, 29.7627) radius 1.35 projected
  circle A524 centre (49.9367, 19.7627) radius 1.35 projected
  circle A525 centre (49.9367, 19.7627) radius 1.35 projected
  circle A526 centre (39.9367, 29.7627) radius 1.35 projected
  circle A527 centre (29.9367, 19.7627) radius 1.35 projected
  circle A528 centre (49.9367, 29.7627) radius 1.35 projected
  circle A529 centre (49.9367, 29.7627) radius 1.35 projected
  circle A530 centre (39.9367, 19.7627) radius 1.35 projected
  circle A531 centre (39.9367, 19.7627) radius 1.35 projected
  circle A532 centre (49.9367, 29.7627) radius 1.35 projected
  circle A533 centre (49.9367, 29.7627) radius 1.35 projected
  circle A534 centre (39.9367, 29.7627) radius 1.35 projected
  circle A535 centre (39.9367, 29.7627) radius 1.35 projected
  circle A536 centre (29.9367, 29.7627) radius 1.35 projected
  circle A537 centre (29.9367, 29.7627) radius 1.35 projected
  circle A538 centre (55.9367, 35.7627) radius 4 projected
  circle A539 centre (55.9367, 35.7627) radius 4 projected
  circle A540 centre (55.9367, 35.7627) radius 4 projected
  circle A541 centre (55.9367, 35.7627) radius 6 projected
  circle A542 centre (55.9367, 35.7627) radius 6 projected
  arc A543 (55.9367, 29.7627) -> (49.9367, 35.7627) centre (55.9367, 35.7627) ccw projected
  arc A544 (49.9367, 35.7627) -> (55.9367, 29.7627) centre (55.9367, 35.7627) ccw projected
  circle A545 centre (55.9367, 35.7627) radius 4 projected
  circle A546 centre (55.9367, 35.7627) radius 6 projected
  circle A547 centre (29.9367, 19.7627) radius 1.35 projected
  circle A548 centre (29.9367, 19.7627) radius 1.35 projected
  circle A549 centre (49.9367, 9.7627) radius 1.35 projected
  point P0 (0, 0)
  point P1 (-56.0633, -0.2373)
  point P2 (55.9367, -0.2373)
  point P3 (3.2533, -36.2373)
  dimension "d33" = 5
  dimension "d34" = 12
  dimension "d35" = 5
  dimension "d36" = 5
  dimension "d37" = 5
  dimension "d38" = 12
  dimension "d39" = 12
  dimension "d40" = 12
  constraints: 20 end point, 17 point on line, 8 point on circle, 4 centre point, 4 coincident, 4 tangent, 3 midpoint, 3 perpendicular, 1 parallel, 1 vertical, 5 other
  measures "d33" distance of L1.start L1.end
  measures "d34" diameter of A0
  measures "d35" distance from line of point (-0.063, 40.763) L2
  measures "d36" distance from line of L3 point (-61.063, -0.237)
  measures "d37" distance from line of point (60.937, -0.237) L4
  measures "d38" diameter of A1
  measures "d39" diameter of A2
  measures "d40" diameter of A3
extrude "Extrusion5" add sketch "Sketch5" against normal up to surface (4 mm away) contours L0 A0 L9 | A0 L0 | L8 A3 L3 | A0 L0 L10 | A3 L3 | A3 L7 L3 | L4 A1 L5 | L4 A1 | L11 A2 L2 | L4 L6 A1 | A2 L2 | A2 L12 L2 picked at (-0.0633, -43.5415) picked at (-60.1175, 1.525) picked at (59.7251, -0.7321) picked at (1.9367, 38.8712)
sketch "Sketch6" plane through (0, 0, 0) normal (0, -1, 0) x (1, 0, 0)
  arc A0 (-61.0633, 6.2373) -> (-61.0633, -5.7627) centre (-61.0633, 0.2373) ccw projected
  circle A1 centre (-61.0633, 0.2373) radius 3
  arc A2 (-6.0633, -40.7627) -> (5.9367, -40.7627) centre (-0.0633, -40.7627) ccw projected
  circle A3 centre (-0.0633, -40.7627) radius 3
  arc A4 (60.9367, -5.7627) -> (60.9367, 6.2373) centre (60.9367, 0.2373) ccw projected
  circle A5 centre (60.9367, 0.2373) radius 3
  arc A6 (5.9367, 41.2373) -> (-6.0633, 41.2373) centre (-0.0633, 41.2373) ccw projected
  circle A7 centre (-0.0633, 41.2373) radius 3
  circle A8 centre (-0.0633, 41.2373) radius 2.1
  circle A9 centre (60.9367, 0.2373) radius 2.1
  circle A10 centre (-0.0633, -40.7627) radius 2.1
  circle A11 centre (-61.0633, 0.2373) radius 2.1
  point P0 (0, 0)
  dimension "d43" = 6
  dimension "d44" = 6
  dimension "d45" = 6
  dimension "d46" = 6
  dimension "d47" = 4.2
  dimension "d48" = 4.2
  dimension "d49" = 4.2
  dimension "d50" = 4.2
  constraints: 8 centre point, 8 coincident
  measures "d43" diameter of A1
  measures "d44" diameter of A3
  measures "d45" diameter of A5
  measures "d46" diameter of A7
  measures "d47" diameter of A8
  measures "d48" diameter of A9
  measures "d49" diameter of A10
  measures "d50" diameter of A11
extrude "Extrusion6" cut sketch "Sketch6" against normal blind 10 contours A1 | A3 | A5 | A7 | A8 | A9 | A10 | A11
fillet "Fillet1" radius 11.525 16 edges at (-50.0633, 2, 36.2373) (5.9367, 2, 36.2373) (49.9367, 2, 36.2373) (-6.0633, 2, 36.2373) (-56.0633, 2, 30.2373) (-56.0633, 2, 6.2373) (-56.0633, 2, -5.7627) (-56.0633, 2, -29.7627) (-50.0633, 2, -35.7627) (-6.0633, 2, -35.7627) (5.9367, 2, -35.7627) (49.9367, 2, -35.7627) (55.9367, 2, -29.7627) (55.9367, 2, -5.7627) (55.9367, 2, 6.2373) (55.9367, 2, 30.2373)
body "Solid1"
